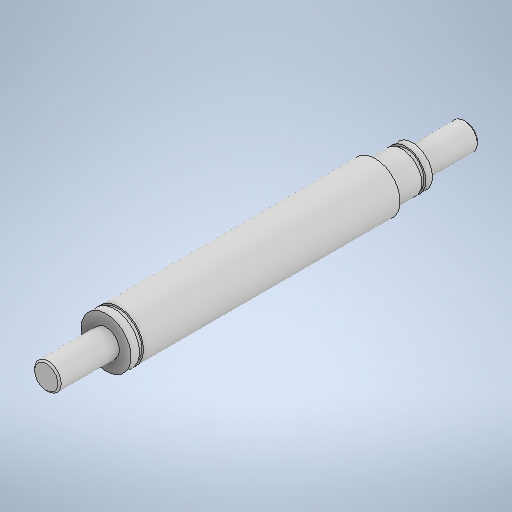
# Autodesk Inventor part: 59-01-002-A
Saved by Autodesk Inventor 2025.2 (Build 292293000, 293)
## iProperties
Created: 2024-11-13
Part Number: 59-01-002-A
Material: Generic
Document SubType Name: Modeling
Designer: Zvonko.Gabric
Density: 1 g/cm^3
Appearance: Default
Author: Zvonko.Gabric
Autodesk Inventor part; units mm, degrees
ref_plane "YZ Plane" through (0, 0, 0) normal (1, 0, 0) x (0, 1, 0)
ref_plane "XZ Plane" through (0, 0, 0) normal (0, 1, 0) x (-1, 0, 0)
ref_plane "XY Plane" through (0, 0, 0) normal (0, 0, 1) x (1, 0, 0)
sketch "Sketch1" plane through (0, 0, 0) normal (0, 1, 0) x (-1, 0, 0)
  line L0 (0, 0) -> (3.5, 0)
  line L1 (4, -0.5) -> (4, -18)
  line L2 (4, -18) -> (7.5, -18)
  line L3 (7.5, -18) -> (7.5, -20.5)
  line L4 (7.5, -20.5) -> (7, -20.5)
  line L5 (7, -20.5) -> (7, -21.7)
  line L6 (7, -21.7) -> (7.5, -21.7)
  line L7 (7.5, -21.7) -> (7.5, -98.8)
  line L8 (7.5, -98.8) -> (6, -98.8)
  line L9 (6, -98.8) -> (6, -106.8)
  line L10 (6, -106.8) -> (5.5, -106.8)
  line L11 (5.5, -106.8) -> (5.5, -108)
  line L12 (5.5, -108) -> (6, -108)
  line L13 (6, -108) -> (6, -110)
  line L14 (6, -110) -> (4, -110)
  line L15 (4, -110) -> (4, -125.5)
  line L16 (4, -125.5) -> (3.5, -126)
  line L17 (3.5, -126) -> (0, -126)
  line L18 (0, 0) -> (0, -126)
  line L19 (4, -0.5) -> (3.5, 0)
  point P0 (5.5, -107.4)
  point P1 (1.75, 0)
  point P2 (5.75, -18)
  point P3 (7.25, -21.7)
  dimension "d2" = 7.5
  dimension "d3" = 2.5
  dimension "d4" = 7.5
  dimension "d6" = 8
  dimension "d8" = 1.5
  dimension "d10" = 1.2
  dimension "d11" = 2
  dimension "d13" = 16
  dimension "d14" = 126
  dimension "d15" = 0.5
  dimension "d16" = 6
  dimension "d18" = 5.5
  dimension "d19" = 1.5
  dimension "d20" = 4
  dimension "d21" = 3.5
  dimension "d22" = 45
  dimension "d23" = 3.5
  dimension "d24" = 0.5
  dimension "d25" = 45
  dimension "d26" = 18
  dimension "d27" = 3.7
  constraints: 40 end point, 10 perpendicular, 5 horizontal, 4 midpoint, 2 vertical
  measures "d2" distance from line of L3 L0.start
  measures "d3" distance of L2.end L3.end
  measures "d4" distance from line of L0.start L7
  measures "d6" distance of L8.end L9.end
  measures "d8" distance of L7.end L8.end
  measures "d10" distance of L10.end L11.end
  measures "d11" distance of L12.end L13.end
  measures "d13" distance between parallel lines of L17 L14
  measures "d14" distance between parallel lines of L17 L0
  measures "d15" distance between parallel lines of L3 L5
  measures "d16" distance from line of L17.end L9
  measures "d18" distance from line of L18 point (5.5, -107.4)
  measures "d19" distance between parallel lines of L7 L13
  measures "d20" distance between parallel lines of L18 L15
  measures "d21" distance of L16.end L17.end
  measures "d22" angle of L17 L16
  measures "d23" distance of L0.start L0.end
  measures "d24" horizontal distance of L1.start L0.end
  measures "d25" angle of L19 L0
  measures "d26" vertical distance of point (1.75, 0) point (5.75, -18)
  measures "d27" distance from line of L2 point (7.25, -21.7)
revolve "Revolution1" add sketch "Sketch1" angle 360 about axis through (0, 0, 0) along (0, 0, -1)
body "Solid1"
